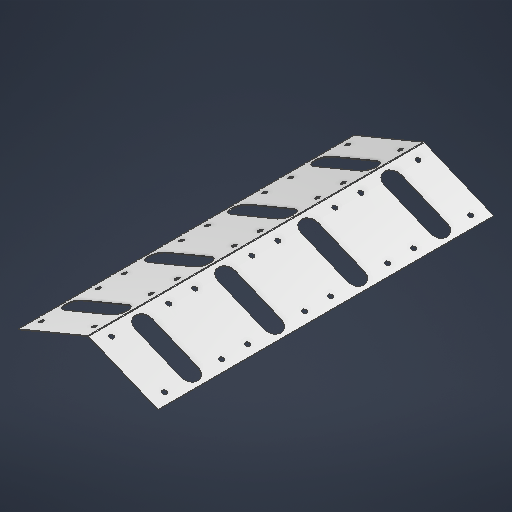
# Autodesk Inventor part: DMF 01 11 cylinder sheet cap v2.1
Saved by Autodesk Inventor 2026.2 (Build 302298010, 298A)
## iProperties
Created: 2024-04-28
Part Number: DMF 01 11 cylinder sheet cap v2.1
Material: Stainless Steel AISI 304
Document SubType Name: Sheet Metal
Designer: pokla
Density: 8 g/cm^3
Appearance: Chrome - Satin
Sheet Metal Rule: Default
Sheet Metal Width: 436,215 mm
Sheet Metal Length: 970,000 mm
Sheet Metal Area: 423128,176 mm^2
Flat Pattern Width: 43.6215 cm
Flat Pattern Length: 97 cm
Flat Pattern Area: 4231.28 cm^2
Stock Number: Барабан_Лист_Крышка
d192: 145,000 mm
d193: 50,000 mm
Author: pokla
Autodesk Inventor part; units mm, degrees
ref_plane "YZ Plane" through (0, 0, 0) normal (1, 0, 0) x (0, 1, 0)
ref_plane "XZ Plane" through (0, 0, 0) normal (0, 1, 0) x (-1, 0, 0)
ref_plane "XY Plane" through (0, 0, 0) normal (0, 0, 1) x (1, 0, 0)
sketch "Sketch1" plane through (0, 0, 0) normal (0, 0, 1) x (1, 0, 0)
  line L0 (-202.822219, 202.822219) -> (0, 286.833933) construction
  line L1 (0, 286.833933) -> (202.822219, 202.822219) construction
  line L2 (202.822219, 202.822219) -> (286.833933, 0) construction
  line L3 (286.833933, 0) -> (202.822219, -202.822219) construction
  line L4 (202.822219, -202.822219) -> (0, -286.833933) construction
  line L5 (0, -286.833933) -> (-202.822219, -202.822219) construction
  line L6 (-202.822219, -202.822219) -> (-286.833933, 0) construction
  line L7 (-286.833933, 0) -> (-202.822219, 202.822219) construction
  line L8 (1.530734, 286.199882) -> (201.990728, 203.166634)
  line L9 (-1.530734, 286.199882) -> (-201.990728, 203.166634)
  arc A0 (1.530734, 286.199882) -> (-1.530734, 286.199882) centre (0, 282.504364) ccw
  point P0 (0, 0)
  point P1 (0, 0)
  dimension "d46" = 530
  dimension "d47" = 0.9
  dimension "d48" = 4
  measures "d46" distance between parallel lines of L7 L3
  measures "d47" distance of L0.start L9.end
  measures "d48" radius of A0
contour flange "Contour Flange2" sketch "Sketch1" thickness 2 bend radius 2 width 970 along (0, 0, -1) mid plane no both sides no wall seen from (101.760731, 244.683258, 0) lies toward (-0.3826834, -0.9238795, 0) curves L8 A0 L9
bend "Bend4"
corner "Corner4"
sketch "Sketch14" plane through (1.530734, 286.199882, 0) normal (0.3826834, 0.9238795, 0) x (0.9238795, -0.3826834, 0)
  line L0 (180.988167, 150) -> (180.988167, 100) construction
  line L1 (180.988167, 100) -> (35.988167, 100)
  line L2 (35.988167, 100) -> (35.988167, 150) construction
  line L3 (35.988167, 150) -> (180.988167, 150)
  circle A0 centre (190.988167, 207.5) radius 6.5
  circle A1 centre (25.988167, 207.5) radius 6.5
  line L4 (108.488167, 100) -> (108.488167, 150) construction
  line L5 (216.976334, 0) -> (0, 0)
  line L6 (108.488167, 125) -> (180.988167, 125) construction
  circle A2 centre (25.988167, 42.5) radius 6.5
  circle A3 centre (190.988167, 42.5) radius 6.5
  arc A4 (180.988167, 100) -> (180.988167, 150) centre (180.988167, 125) ccw
  arc A5 (35.988167, 150) -> (35.988167, 100) centre (35.988167, 125) ccw
  point P0 (108.488167, 0)
  dimension "d163" = 13
  dimension "d164" = 145
  dimension "d165" = 50
  dimension "d167" = 165
  dimension "d171" = 100
  dimension "d181" = 165
  constraints: 12 end point, 6 centre point, 5 midpoint, 4 point on circle, 4 tangent, 2 parallel, 1 perpendicular, 1 vertical alignment, 3 other
  measures "d163" diameter of A0
  measures "d164" distance of L2.end L0.start
  measures "d165" distance of L0.start L0.end
  measures "d167" distance of A1.centre A0.centre
  measures "d171" distance between parallel lines of L5 L1
  measures "d181" distance of A1.centre A2.centre
extrude "Cut2" cut sketch "Sketch14" against normal through all
pattern_linear "Rectangular Pattern7" count 4 spacing 240 along (0, 0, -1) of "Cut2"
pattern_circular "Circular Pattern2" count 2 over 45 about axis through (0, 0, -10) along (0, 0, 1) of "Cut2", "Rectangular Pattern7"
equation "\"d46\" = Барабан_размер_по_плоскостям"
equation "\"d47\" = Барабан_отступ_развертки"
equation "\"d48\" = BendRadius + Thickness"
equation "\"d49\" = Thickness"
equation "\"d50\" = BendReliefWidth"
equation "\"d51\" = BendReliefDepth"
equation "\"d52\" = MinimumRemnant"
equation "\"d53\" = TransitionRadius"
equation "\"d55\" = BendRadius"
equation "\"d57\" = CornerReliefSize"
equation "\"d58\" = GapSize"
equation "\"d59\" = JacobiRadiusSize"
equation "\"BendRadius\" = Thickness"
equation "\"BendReliefWidth\" = Thickness"
equation "\"BendReliefDepth\" = 0.5 * Thickness"
equation "\"CornerReliefSize\" = 4 * Thickness"
equation "\"MinimumRemnant\" = 2 * Thickness"
equation "\"TransitionRadius\" = BendRadius"
equation "\"JacobiRadiusSize\" = BendRadius"
equation "\"GapSize\" = Thickness"
equation "\"d192\" = 145"
equation "\"Барабан_размер_по_плоскостям\" = 530"
equation "\"Барабан_отступ_развертки\" = 0.9"
equation "\"Thickness\" = 2"
body "Solid2"
